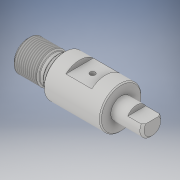
# Autodesk Inventor part: Вал
Saved by Autodesk Inventor 2019.3 (Build 233278000, 278)
## iProperties
Created: 2020-04-03
Part Number: Вал
Material: Типовые
Document SubType Name: Modeling
Designer: Admin
Density: 1 g/cm^3
Appearance: По умолчанию
Mass: 98.5821 g
Surface Area: 147.635 cm^2
Volume: 98.5821 cm^3
Author: Admin
Autodesk Inventor part; units mm, degrees
ref_plane "YZ Plane" through (0, 0, 0) normal (1, 0, 0) x (0, 1, 0)
ref_plane "XZ Plane" through (0, 0, 0) normal (0, 1, 0) x (-1, 0, 0)
ref_plane "XY Plane" through (0, 0, 0) normal (0, 0, 1) x (1, 0, 0)
sketch "Эскиз1" plane through (0, 0, 0) normal (0, 1, 0) x (-1, 0, 0)
  line L0 (0, 0) -> (0, -15)
  line L1 (0, -15) -> (-23.5, -15)
  line L2 (-23.5, -15) -> (-24.7071, -13.7929)
  line L3 (-25.4142, -13.5) -> (-28.4, -13.5)
  line L4 (-35, -20) -> (-90, -20)
  line L5 (-90, -20) -> (-90, -10)
  line L6 (-90, -10) -> (-120, -10)
  line L7 (-120, -10) -> (-120, 0)
  line L8 (-30, -15.1) -> (-30, -15)
  line L9 (-30, -15) -> (-35, -15)
  line L10 (-35, -15) -> (-35, -20)
  line L11 (0, 0) -> (-120, 0)
  line L12 (24, 0) -> (-144, 0) projected
  arc A0 (-24.7071, -13.7929) -> (-25.4142, -13.5) centre (-25.4142, -14.5) ccw
  arc A1 (-28.4, -13.5) -> (-30, -15.1) centre (-28.4, -15.1) ccw
  point P0 (-25, -13.5)
  point P1 (-30, -13.5)
  dimension "d3" = 45
  dimension "d6" = 5
  dimension "d8" = 30
  dimension "d9" = 35
  dimension "d11" = 55
  dimension "d14" = 15
  dimension "d15" = 13.5
  dimension "d16" = 15
  dimension "d17" = 20
  dimension "d18" = 10
  dimension "d19" = 120
  dimension "d20" = 1
  dimension "d21" = 1.6
  constraints: 24 end point, 6 horizontal, 5 vertical, 4 point on circle, 4 point on line, 4 tangent, 2 centre point, 1 horizontal alignment
  measures "d3" angle of L1 L2
  measures "d6" distance of point (-30, -13.5) point (-25, -13.5)
  measures "d8" distance from line of L0 point (-30, -13.5)
  measures "d9" distance between parallel lines of L0 L10
  measures "d11" distance between parallel lines of L10 L5
  measures "d14" distance between parallel lines of L11 L1
  measures "d15" distance between parallel lines of L11 L3
  measures "d16" distance between parallel lines of L11 L9
  measures "d17" distance between parallel lines of L11 L4
  measures "d18" distance between parallel lines of L11 L6
  measures "d19" distance between parallel lines of L0 L7
  measures "d20" radius of A0
  measures "d21" radius of A1
revolve "Вращение1" add sketch "Эскиз1" angle 360 about axis through (-10, 0, 0) along (1, 0, 0)
thread "Резьба1" size "M30x2" class "6g" standard "ANSI Metric M Profile" full length
chamfer "Фаска1" distance 2 angle 45 2 edges at (0, 0, 15) (120, 0, 10)
chamfer "Фаска2" distance 1 angle 45 2 edges at (35, 0, 20) (90, 0, 20)
sketch "Эскиз2" plane through (0, 0, 0) normal (0, 0, 1) x (1, 0, 0)
  line L0 (105, 10) -> (105, 5)
  line L1 (105, 5) -> (120, 5)
  line L2 (120, 5) -> (120, 10)
  line L3 (120, 10) -> (105, 10)
  line L4 (120, 8) -> (120, -8) projected
  line L5 (90, 10) -> (118, 10) projected
  line L6 (90, -10) -> (118, -10) projected
  point P0 (0, 0)
  dimension "d30" = 15
  dimension "d31" = 15
  constraints: 8 end point, 2 horizontal, 2 vertical, 1 horizontal alignment, 1 vertical alignment
  measures "d30" distance between parallel lines of L2 L0
  measures "d31" distance between parallel lines of L6 L1
extrude "Выдавливание1" cut sketch "Эскиз2" along normal through all both and the other way through all
sketch "Эскиз3" plane through (0, 0, 0) normal (0, 0, 1) x (1, 0, 0)
  line L0 (50, 20) -> (50, 15)
  line L1 (50, 15) -> (75, 15)
  line L2 (75, 15) -> (75, 20)
  line L3 (75, 20) -> (50, 20)
  line L4 (35, -19) -> (35, 19) projected
  line L5 (36, 20) -> (89, 20) projected
  line L6 (36, -20) -> (89, -20) projected
  point P0 (0, 0)
  dimension "d34" = 35
  dimension "d35" = 15
  dimension "d36" = 25
  constraints: 8 end point, 2 horizontal, 2 vertical, 1 horizontal alignment
  measures "d34" distance between parallel lines of L1 L6
  measures "d35" distance between parallel lines of L4 L0
  measures "d36" distance between parallel lines of L2 L0
extrude "Выдавливание2" cut sketch "Эскиз3" along normal through all both and the other way through all
sketch "Эскиз4" plane through (50, 15, -13.2288) normal (0, 1, 0) x (1, 0, 0)
  line L0 (-74, -13.2288) -> (94, -13.2288) projected
  line L1 (0, 0) -> (0, -26.4575) projected
  point P0 (-50, -13.2288)
  point P1 (12.5, -13.2288)
  dimension "d39" = 12.5
  constraints: 1 point on line
  measures "d39" distance from line of L1 point (12.5, -13.229)
hole "Отверстие1" at (62.5, 15, 0) direction (0, -1, 0) diameter 5 depth 20 tip angle 120
